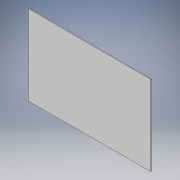
# Autodesk Inventor part: NorthWall
Saved by Autodesk Inventor 2018 (Build 220112000, 112)
## iProperties
Created: 2019-04-28
Part Number: NorthWall
Material: Generic
Document SubType Name: Modeling
Designer: snipe
Density: 1 g/cm^3
Appearance: Default
Author: snipe
Autodesk Inventor part; units mm, degrees
ref_plane "YZ Plane" through (0, 0, 0) normal (1, 0, 0) x (0, 1, 0)
ref_plane "XZ Plane" through (0, 0, 0) normal (0, 1, 0) x (-1, 0, 0)
ref_plane "XY Plane" through (0, 0, 0) normal (0, 0, 1) x (1, 0, 0)
sketch "Sketch1" plane through (0, 0, 0) normal (0, 0, 1) x (1, 0, 0)
  line L0 (0, 1813.56) -> (0, -1813.56) projected
  line L1 (-2773.68, 0) -> (2773.68, 0) projected
  line L2 (0, -1813.56) -> (0, 1813.56) projected
  line L3 (-2773.68, 0) -> (2773.68, 0) projected
  line L4 (-1981.2, -1295.4) -> (1981.2, -1295.4)
  line L5 (1981.2, -1295.4) -> (1981.2, 1295.4)
  line L6 (1981.2, 1295.4) -> (-1981.2, 1295.4)
  line L7 (-1981.2, 1295.4) -> (-1981.2, -1295.4)
  point P0 (0, 0)
  dimension "d0" = 3962.4
  dimension "d1" = 2590.8
  constraints: 8 end point, 2 parallel, 1 horizontal, 1 perpendicular, 2 other
  measures "d0" distance of L6.end L5.end
  measures "d1" distance of L5.end L4.end
extrude "Extrusion1" add sketch "Sketch1" along normal blind 25.4
body "Solid1"
